Autodesk Inventor part; units mm, degrees
(part 2 of 6)
  line L866 (-45.2872, 131.2388) -> (-45.0362, 131.5916)
  line L867 (-45.0362, 131.5916) -> (-44.769, 131.9317)
  line L868 (-44.769, 131.9317) -> (-44.4862, 132.2582)
  line L869 (-44.4862, 132.2582) -> (-44.1882, 132.5707)
  line L870 (-44.1882, 132.5707) -> (-43.8757, 132.8687)
  line L871 (-43.8757, 132.8687) -> (-43.5491, 133.1516)
  line L872 (-43.5491, 133.1516) -> (-43.2091, 133.4189)
  line L873 (-43.2091, 133.4189) -> (-42.8561, 133.6697)
  line L874 (-42.8561, 133.6697) -> (-42.4911, 133.904)
  line L875 (-42.4911, 133.904) -> (-42.1142, 134.1207)
  line L876 (-42.1142, 134.1207) -> (-41.7261, 134.3194)
  line L877 (-41.7261, 134.3194) -> (-41.3274, 134.4996)
  line L878 (-41.3274, 134.4996) -> (-40.9188, 134.6609)
  line L879 (-40.9188, 134.6609) -> (-40.5005, 134.8021)
  line L880 (-40.5005, 134.8021) -> (-40.0735, 134.9234)
  line L881 (-40.0735, 134.9234) -> (-39.6381, 135.024)
  line L882 (-39.6381, 135.024) -> (-39.1949, 135.1032)
  line L883 (-39.1949, 135.1032) -> (-38.7444, 135.1604)
  line L884 (-38.7444, 135.1604) -> (-38.2874, 135.1952)
  line L885 (-38.2874, 135.1952) -> (-37.8242, 135.2069)
  line L886 (-37.8242, 135.2069) -> (-37.361, 135.1952)
  line L887 (-37.361, 135.1952) -> (-36.904, 135.1604)
  line L888 (-36.904, 135.1604) -> (-36.4536, 135.1032)
  line L889 (-36.4536, 135.1032) -> (-36.0104, 135.024)
  line L890 (-36.0104, 135.024) -> (-35.5749, 134.9234)
  line L891 (-35.5749, 134.9234) -> (-35.1479, 134.8021)
  line L892 (-35.1479, 134.8021) -> (-34.7297, 134.6609)
  line L893 (-34.7297, 134.6609) -> (-34.3211, 134.4996)
  line L894 (-34.3211, 134.4996) -> (-33.9223, 134.3194)
  line L895 (-33.9223, 134.3194) -> (-33.5342, 134.1207)
  line L896 (-33.5342, 134.1207) -> (-33.1573, 133.904)
  line L897 (-33.1573, 133.904) -> (-32.7923, 133.6697)
  line L898 (-32.7923, 133.6697) -> (-32.4394, 133.4189)
  line L899 (-32.4394, 133.4189) -> (-32.0993, 133.1516)
  line L900 (-32.0993, 133.1516) -> (-31.7729, 132.8687)
  line L901 (-31.7729, 132.8687) -> (-31.4603, 132.5707)
  line L902 (-31.4603, 132.5707) -> (-31.1623, 132.2582)
  line L903 (-31.1623, 132.2582) -> (-30.8794, 131.9317)
  line L904 (-30.8794, 131.9317) -> (-30.6123, 131.5916)
  line L905 (-30.6123, 131.5916) -> (-30.3613, 131.2388)
  line L906 (-30.3613, 131.2388) -> (-30.1272, 130.8737)
  line L907 (-30.1272, 130.8737) -> (-29.9105, 130.4968)
  line L908 (-29.9105, 130.4968) -> (-29.7117, 130.1089)
  line L909 (-29.7117, 130.1089) -> (-29.5315, 129.7099)
  line L910 (-29.5315, 129.7099) -> (-29.3703, 129.3013)
  line L911 (-29.3703, 129.3013) -> (-29.2289, 128.8831)
  line L912 (-29.2289, 128.8831) -> (-29.1076, 128.4559)
  line L913 (-29.1076, 128.4559) -> (-29.007, 128.0208)
  line L914 (-29.007, 128.0208) -> (-28.928, 127.5774)
  line L915 (-28.928, 127.5774) -> (-28.8708, 127.1271)
  line L916 (-28.8708, 127.1271) -> (-28.836, 126.67)
  line L917 (-28.836, 126.67) -> (-28.8243, 126.2069)
  line L918 (-28.8243, 126.2069) -> (-28.836, 125.7436)
  line L919 (-28.836, 125.7436) -> (-28.8708, 125.2868)
  line L920 (-28.8708, 125.2868) -> (-28.928, 124.8361)
  line L921 (-28.928, 124.8361) -> (-29.007, 124.3931)
  line L922 (-29.007, 124.3931) -> (-29.1076, 123.9576)
  line L923 (-29.1076, 123.9576) -> (-29.2289, 123.5304)
  line L924 (-29.2289, 123.5304) -> (-29.3703, 123.1122)
  line L925 (-29.3703, 123.1122) -> (-29.5315, 122.7036)
  line L926 (-29.5315, 122.7036) -> (-29.7117, 122.305)
  line L927 (-29.7117, 122.305) -> (-29.9105, 121.9168)
  line L928 (-29.9105, 121.9168) -> (-30.1272, 121.5399)
  line L929 (-30.1272, 121.5399) -> (-30.3613, 121.1747)
  line L930 (-30.3613, 121.1747) -> (-30.6123, 120.8219)
  line L931 (-30.6123, 120.8219) -> (-30.8794, 120.4819)
  line L932 (-30.8794, 120.4819) -> (-31.1623, 120.1553)
  line L933 (-31.1623, 120.1553) -> (-31.4603, 119.8428)
  line L934 (-31.4603, 119.8428) -> (-31.7729, 119.5448)
  line L935 (-31.7729, 119.5448) -> (-32.0993, 119.262)
  line L936 (-32.0993, 119.262) -> (-32.4394, 118.995)
  line L937 (-32.4394, 118.995) -> (-32.7923, 118.7438)
  line L938 (-32.7923, 118.7438) -> (-33.1573, 118.5099)
  line L939 (-33.1573, 118.5099) -> (-33.5342, 118.2932)
  line L940 (-33.5342, 118.2932) -> (-33.9223, 118.0944)
  line L941 (-33.9223, 118.0944) -> (-34.3211, 117.9142)
  line L942 (-34.3211, 117.9142) -> (-34.7297, 117.753)
  line L943 (-34.7297, 117.753) -> (-35.1479, 117.6114)
  line L944 (-35.1479, 117.6114) -> (-35.5749, 117.4902)
  line L945 (-35.5749, 117.4902) -> (-36.0104, 117.3896)
  line L946 (-36.0104, 117.3896) -> (-36.4536, 117.3107)
  line L947 (-36.4536, 117.3107) -> (-36.904, 117.2531)
  line L948 (-36.904, 117.2531) -> (-37.361, 117.2187)
  line L949 (-37.361, 117.2187) -> (-37.8242, 117.207)
  line L950 (-37.8242, 117.207) -> (-38.2874, 117.2187)
  line L951 (-38.2874, 117.2187) -> (-38.7444, 117.2531)
  line L952 (-38.7444, 117.2531) -> (-39.1949, 117.3107)
  line L953 (-39.1949, 117.3107) -> (-39.6381, 117.3896)
  line L954 (-39.6381, 117.3896) -> (-40.0735, 117.4902)
  line L955 (-40.0735, 117.4902) -> (-40.5005, 117.6114)
  line L956 (-40.5005, 117.6114) -> (-40.9188, 117.753)
  line L957 (-40.9188, 117.753) -> (-41.3274, 117.9142)
  line L958 (-41.3274, 117.9142) -> (-41.7261, 118.0944)
  line L959 (-41.7261, 118.0944) -> (-42.1142, 118.2932)
  line L960 (-42.1142, 118.2932) -> (-42.4911, 118.5099)
  line L961 (-42.4911, 118.5099) -> (-42.8561, 118.7438)
  line L962 (-42.8561, 118.7438) -> (-43.2091, 118.995)
  line L963 (-43.2091, 118.995) -> (-43.5491, 119.262)
  line L964 (-43.5491, 119.262) -> (-43.8757, 119.5448)
  line L965 (-43.8757, 119.5448) -> (-44.1882, 119.8428)
  line L966 (-44.1882, 119.8428) -> (-44.4862, 120.1553)
  line L967 (-44.4862, 120.1553) -> (-44.769, 120.4819)
  line L968 (-44.769, 120.4819) -> (-45.0362, 120.8219)
  line L969 (-45.0362, 120.8219) -> (-45.2872, 121.1747)
  line L970 (-45.2872, 121.1747) -> (-45.5213, 121.5399)
  line L971 (-45.5213, 121.5399) -> (-45.7379, 121.9168)
  line L972 (-45.7379, 121.9168) -> (-45.9367, 122.305)
  line L973 (-45.9367, 122.305) -> (-46.1169, 122.7036)
  line L974 (-46.1169, 122.7036) -> (-46.2781, 123.1122)
  line L975 (-46.2781, 123.1122) -> (-46.4196, 123.5304)
  line L976 (-46.4196, 123.5304) -> (-46.5408, 123.9576)
  line L977 (-46.5408, 123.9576) -> (-46.6414, 124.3931)
  line L978 (-46.6414, 124.3931) -> (-46.7205, 124.8361)
  line L979 (-46.7205, 124.8361) -> (-46.7777, 125.2868)
  line L980 (-46.7777, 125.2868) -> (-46.8125, 125.7436)
  line L981 (-46.8125, 125.7436) -> (-46.8242, 126.2069)
  line L982 (-46.8338, 98.1969) -> (-46.8221, 98.66)
  line L983 (-46.8221, 98.66) -> (-46.7873, 99.1171)
  line L984 (-46.7873, 99.1171) -> (-46.7301, 99.5674)
  line L985 (-46.7301, 99.5674) -> (-46.6511, 100.0108)
  line L986 (-46.6511, 100.0108) -> (-46.5505, 100.4462)
  line L987 (-46.5505, 100.4462) -> (-46.4292, 100.8731)
  line L988 (-46.4292, 100.8731) -> (-46.2878, 101.2913)
  line L989 (-46.2878, 101.2913) -> (-46.1266, 101.6999)
  line L990 (-46.1266, 101.6999) -> (-45.9464, 102.0988)
  line L991 (-45.9464, 102.0988) -> (-45.7476, 102.4868)
  line L992 (-45.7476, 102.4868) -> (-45.5309, 102.8637)
  line L993 (-45.5309, 102.8637) -> (-45.2968, 103.2288)
  line L994 (-45.2968, 103.2288) -> (-45.0458, 103.5816)
  line L995 (-45.0458, 103.5816) -> (-44.7787, 103.9216)
  line L996 (-44.7787, 103.9216) -> (-44.4958, 104.2482)
  line L997 (-44.4958, 104.2482) -> (-44.1978, 104.5607)
  line L998 (-44.1978, 104.5607) -> (-43.8852, 104.8587)
  line L999 (-43.8852, 104.8587) -> (-43.5588, 105.1416)
  line L1000 (-43.5588, 105.1416) -> (-43.2187, 105.4089)
  line L1001 (-43.2187, 105.4089) -> (-42.8658, 105.6597)
  line L1002 (-42.8658, 105.6597) -> (-42.5008, 105.894)
  line L1003 (-42.5008, 105.894) -> (-42.1239, 106.1107)
  line L1004 (-42.1239, 106.1107) -> (-41.7358, 106.3094)
  line L1005 (-41.7358, 106.3094) -> (-41.337, 106.4896)
  line L1006 (-41.337, 106.4896) -> (-40.9284, 106.6509)
  line L1007 (-40.9284, 106.6509) -> (-40.5102, 106.7921)
  line L1008 (-40.5102, 106.7921) -> (-40.0832, 106.9134)
  line L1009 (-40.0832, 106.9134) -> (-39.6477, 107.014)
  line L1010 (-39.6477, 107.014) -> (-39.2045, 107.0932)
  line L1011 (-39.2045, 107.0932) -> (-38.7541, 107.1504)
  line L1012 (-38.7541, 107.1504) -> (-38.2971, 107.1852)
  line L1013 (-38.2971, 107.1852) -> (-37.8339, 107.1969)
  line L1014 (-37.8339, 107.1969) -> (-37.3707, 107.1852)
  line L1015 (-37.3707, 107.1852) -> (-36.9137, 107.1504)
  line L1016 (-36.9137, 107.1504) -> (-36.4632, 107.0932)
  line L1017 (-36.4632, 107.0932) -> (-36.02, 107.014)
  line L1018 (-36.02, 107.014) -> (-35.5846, 106.9134)
  line L1019 (-35.5846, 106.9134) -> (-35.1575, 106.7921)
  line L1020 (-35.1575, 106.7921) -> (-34.7393, 106.6509)
  line L1021 (-34.7393, 106.6509) -> (-34.3307, 106.4896)
  line L1022 (-34.3307, 106.4896) -> (-33.932, 106.3094)
  line L1023 (-33.932, 106.3094) -> (-33.5439, 106.1107)
  line L1024 (-33.5439, 106.1107) -> (-33.167, 105.894)
  line L1025 (-33.167, 105.894) -> (-32.8018, 105.6597)
  line L1026 (-32.8018, 105.6597) -> (-32.449, 105.4089)
  line L1027 (-32.449, 105.4089) -> (-32.109, 105.1416)
  line L1028 (-32.109, 105.1416) -> (-31.7824, 104.8587)
  line L1029 (-31.7824, 104.8587) -> (-31.4699, 104.5607)
  line L1030 (-31.4699, 104.5607) -> (-31.1719, 104.2482)
  line L1031 (-31.1719, 104.2482) -> (-30.8891, 103.9216)
  line L1032 (-30.8891, 103.9216) -> (-30.6219, 103.5816)
  line L1033 (-30.6219, 103.5816) -> (-30.3709, 103.2288)
  line L1034 (-30.3709, 103.2288) -> (-30.1368, 102.8637)
  line L1035 (-30.1368, 102.8637) -> (-29.9201, 102.4868)
  line L1036 (-29.9201, 102.4868) -> (-29.7214, 102.0988)
  line L1037 (-29.7214, 102.0988) -> (-29.5412, 101.6999)
  line L1038 (-29.5412, 101.6999) -> (-29.3799, 101.2913)
  line L1039 (-29.3799, 101.2913) -> (-29.2385, 100.8731)
  line L1040 (-29.2385, 100.8731) -> (-29.1173, 100.4462)
  line L1041 (-29.1173, 100.4462) -> (-29.0167, 100.0108)
  line L1042 (-29.0167, 100.0108) -> (-28.9376, 99.5674)
  line L1043 (-28.9376, 99.5674) -> (-28.8802, 99.1171)
  line L1044 (-28.8802, 99.1171) -> (-28.8456, 98.66)
  line L1045 (-28.8456, 98.66) -> (-28.8339, 98.1969)
  line L1046 (-28.8339, 98.1969) -> (-28.8456, 97.7336)
  line L1047 (-28.8456, 97.7336) -> (-28.8802, 97.2767)
  line L1048 (-28.8802, 97.2767) -> (-28.9376, 96.8261)
  line L1049 (-28.9376, 96.8261) -> (-29.0167, 96.3831)
  line L1050 (-29.0167, 96.3831) -> (-29.1173, 95.9476)
  line L1051 (-29.1173, 95.9476) -> (-29.2385, 95.5204)
  line L1052 (-29.2385, 95.5204) -> (-29.3799, 95.1022)
  line L1053 (-29.3799, 95.1022) -> (-29.5412, 94.6936)
  line L1054 (-29.5412, 94.6936) -> (-29.7214, 94.295)
  line L1055 (-29.7214, 94.295) -> (-29.9201, 93.9068)
  line L1056 (-29.9201, 93.9068) -> (-30.1368, 93.5299)
  line L1057 (-30.1368, 93.5299) -> (-30.3709, 93.1647)
  line L1058 (-30.3709, 93.1647) -> (-30.6219, 92.8119)
  line L1059 (-30.6219, 92.8119) -> (-30.8891, 92.4719)
  line L1060 (-30.8891, 92.4719) -> (-31.1719, 92.1453)
  line L1061 (-31.1719, 92.1453) -> (-31.4699, 91.8328)
  line L1062 (-31.4699, 91.8328) -> (-31.7824, 91.5348)
  line L1063 (-31.7824, 91.5348) -> (-32.109, 91.252)
  line L1064 (-32.109, 91.252) -> (-32.449, 90.985)
  line L1065 (-32.449, 90.985) -> (-32.8018, 90.7338)
  line L1066 (-32.8018, 90.7338) -> (-33.167, 90.4999)
  line L1067 (-33.167, 90.4999) -> (-33.5439, 90.2832)
  line L1068 (-33.5439, 90.2832) -> (-33.932, 90.0844)
  line L1069 (-33.932, 90.0844) -> (-34.3307, 89.9042)
  line L1070 (-34.3307, 89.9042) -> (-34.7393, 89.743)
  line L1071 (-34.7393, 89.743) -> (-35.1575, 89.6014)
  line L1072 (-35.1575, 89.6014) -> (-35.5846, 89.4802)
  line L1073 (-35.5846, 89.4802) -> (-36.02, 89.3796)
  line L1074 (-36.02, 89.3796) -> (-36.4632, 89.3007)
  line L1075 (-36.4632, 89.3007) -> (-36.9137, 89.2431)
  line L1076 (-36.9137, 89.2431) -> (-37.3707, 89.2087)
  line L1077 (-37.3707, 89.2087) -> (-37.8339, 89.197)
  line L1078 (-37.8339, 89.197) -> (-38.2971, 89.2087)
  line L1079 (-38.2971, 89.2087) -> (-38.7541, 89.2431)
  line L1080 (-38.7541, 89.2431) -> (-39.2045, 89.3007)
  line L1081 (-39.2045, 89.3007) -> (-39.6477, 89.3796)
  line L1082 (-39.6477, 89.3796) -> (-40.0832, 89.4802)
  line L1083 (-40.0832, 89.4802) -> (-40.5102, 89.6014)
  line L1084 (-40.5102, 89.6014) -> (-40.9284, 89.743)
  line L1085 (-40.9284, 89.743) -> (-41.337, 89.9042)
  line L1086 (-41.337, 89.9042) -> (-41.7358, 90.0844)
  line L1087 (-41.7358, 90.0844) -> (-42.1239, 90.2832)
  line L1088 (-42.1239, 90.2832) -> (-42.5008, 90.4999)
  line L1089 (-42.5008, 90.4999) -> (-42.8658, 90.7338)
  line L1090 (-42.8658, 90.7338) -> (-43.2187, 90.985)
  line L1091 (-43.2187, 90.985) -> (-43.5588, 91.252)
  line L1092 (-43.5588, 91.252) -> (-43.8852, 91.5348)
  line L1093 (-43.8852, 91.5348) -> (-44.1978, 91.8328)
  line L1094 (-44.1978, 91.8328) -> (-44.4958, 92.1453)
  line L1095 (-44.4958, 92.1453) -> (-44.7787, 92.4719)
  line L1096 (-44.7787, 92.4719) -> (-45.0458, 92.8119)
  line L1097 (-45.0458, 92.8119) -> (-45.2968, 93.1647)
  line L1098 (-45.2968, 93.1647) -> (-45.5309, 93.5299)
  line L1099 (-45.5309, 93.5299) -> (-45.7476, 93.9068)
  line L1100 (-45.7476, 93.9068) -> (-45.9464, 94.295)
  line L1101 (-45.9464, 94.295) -> (-46.1266, 94.6936)
  line L1102 (-46.1266, 94.6936) -> (-46.2878, 95.1022)
  line L1103 (-46.2878, 95.1022) -> (-46.4292, 95.5204)
  line L1104 (-46.4292, 95.5204) -> (-46.5505, 95.9476)
  line L1105 (-46.5505, 95.9476) -> (-46.6511, 96.3831)
  line L1106 (-46.6511, 96.3831) -> (-46.7301, 96.8261)
  line L1107 (-46.7301, 96.8261) -> (-46.7873, 97.2767)
  line L1108 (-46.7873, 97.2767) -> (-46.8221, 97.7336)
  line L1109 (-46.8221, 97.7336) -> (-46.8338, 98.1969)
  line L1110 (-3.6981, 170.452) -> (-3.6749, 170.912)
  line L1111 (-3.6749, 170.912) -> (-3.6067, 171.3589)
  line L1112 (-3.6067, 171.3589) -> (-3.4957, 171.7902)
  line L1113 (-3.4957, 171.7902) -> (-3.3445, 172.2036)
  line L1114 (-3.3445, 172.2036) -> (-3.155, 172.5969)
  line L1115 (-3.155, 172.5969) -> (-2.9295, 172.9679)
  line L1116 (-2.9295, 172.9679) -> (-2.6705, 173.3143)
  line L1117 (-2.6705, 173.3143) -> (-2.38, 173.634)
  line L1118 (-2.38, 173.634) -> (-2.0605, 173.9244)
  line L1119 (-2.0605, 173.9244) -> (-1.7141, 174.1835)
  line L1120 (-1.7141, 174.1835) -> (-1.3431, 174.4088)
  line L1121 (-1.3431, 174.4088) -> (-0.9496, 174.5983)
  line L1122 (-0.9496, 174.5983) -> (-0.5362, 174.7497)
  line L1123 (-0.5362, 174.7497) -> (-0.1051, 174.8605)
  line L1124 (-0.1051, 174.8605) -> (0.3418, 174.9287)
  line L1125 (0.3418, 174.9287) -> (0.8018, 174.9519)
  line L1126 (0.8018, 174.9519) -> (1.2619, 174.9287)
  line L1127 (1.2619, 174.9287) -> (1.7088, 174.8605)
  line L1128 (1.7088, 174.8605) -> (2.1401, 174.7497)
  line L1129 (2.1401, 174.7497) -> (2.5535, 174.5983)
  line L1130 (2.5535, 174.5983) -> (2.9469, 174.4088)
  line L1131 (2.9469, 174.4088) -> (3.318, 174.1835)
  line L1132 (3.318, 174.1835) -> (3.6644, 173.9244)
  line L1133 (3.6644, 173.9244) -> (3.9839, 173.634)
  line L1134 (3.9839, 173.634) -> (4.2743, 173.3143)
  line L1135 (4.2743, 173.3143) -> (4.5334, 172.9679)
  line L1136 (4.5334, 172.9679) -> (4.7587, 172.5969)
  line L1137 (4.7587, 172.5969) -> (4.9482, 172.2036)
  line L1138 (4.9482, 172.2036) -> (5.0996, 171.7902)
  line L1139 (5.0996, 171.7902) -> (5.2105, 171.3589)
  line L1140 (5.2105, 171.3589) -> (5.2787, 170.912)
  line L1141 (5.2787, 170.912) -> (5.3018, 170.452)
  line L1142 (5.3018, 170.452) -> (5.2787, 169.9919)
  line L1143 (5.2787, 169.9919) -> (5.2105, 169.545)
  line L1144 (5.2105, 169.545) -> (5.0996, 169.1139)
  line L1145 (5.0996, 169.1139) -> (4.9482, 168.7003)
  line L1146 (4.9482, 168.7003) -> (4.7587, 168.307)
  line L1147 (4.7587, 168.307) -> (4.5334, 167.936)
  line L1148 (4.5334, 167.936) -> (4.2743, 167.5896)
  line L1149 (4.2743, 167.5896) -> (3.9839, 167.2701)
  line L1150 (3.9839, 167.2701) -> (3.6644, 166.9795)
  line L1151 (3.6644, 166.9795) -> (3.318, 166.7206)
  line L1152 (3.318, 166.7206) -> (2.9469, 166.4951)
  line L1153 (2.9469, 166.4951) -> (2.5535, 166.3056)
  line L1154 (2.5535, 166.3056) -> (2.1401, 166.1542)
  line L1155 (2.1401, 166.1542) -> (1.7088, 166.0434)
  line L1156 (1.7088, 166.0434) -> (1.2619, 165.9752)
  line L1157 (1.2619, 165.9752) -> (0.8018, 165.952)
  line L1158 (0.8018, 165.952) -> (0.3418, 165.9752)
  line L1159 (0.3418, 165.9752) -> (-0.1051, 166.0434)
  line L1160 (-0.1051, 166.0434) -> (-0.5362, 166.1542)
  line L1161 (-0.5362, 166.1542) -> (-0.9496, 166.3056)
  line L1162 (-0.9496, 166.3056) -> (-1.3431, 166.4951)
  line L1163 (-1.3431, 166.4951) -> (-1.7141, 166.7206)
  line L1164 (-1.7141, 166.7206) -> (-2.0605, 166.9795)
  line L1165 (-2.0605, 166.9795) -> (-2.38, 167.2701)
  line L1166 (-2.38, 167.2701) -> (-2.6705, 167.5896)
  line L1167 (-2.6705, 167.5896) -> (-2.9295, 167.936)
  line L1168 (-2.9295, 167.936) -> (-3.155, 168.307)
  line L1169 (-3.155, 168.307) -> (-3.3445, 168.7003)
  line L1170 (-3.3445, 168.7003) -> (-3.4957, 169.1139)
  line L1171 (-3.4957, 169.1139) -> (-3.6067, 169.545)
  line L1172 (-3.6067, 169.545) -> (-3.6749, 169.9919)
  line L1173 (-3.6749, 169.9919) -> (-3.6981, 170.452)
  line L1174 (-3.7014, 126.9587) -> (-3.6782, 127.4189)
  line L1175 (-3.6782, 127.4189) -> (-3.6099, 127.8658)
  line L1176 (-3.6099, 127.8658) -> (-3.499, 128.2971)
  line L1177 (-3.499, 128.2971) -> (-3.3478, 128.7105)
  line L1178 (-3.3478, 128.7105) -> (-3.1583, 129.1039)
  line L1179 (-3.1583, 129.1039) -> (-2.9328, 129.475)
  line L1180 (-2.9328, 129.475) -> (-2.6737, 129.8212)
  line L1181 (-2.6737, 129.8212) -> (-2.3833, 130.1409)
  line L1182 (-2.3833, 130.1409) -> (-2.0638, 130.4313)
  line L1183 (-2.0638, 130.4313) -> (-1.7174, 130.6904)
  line L1184 (-1.7174, 130.6904) -> (-1.3463, 130.9157)
  line L1185 (-1.3463, 130.9157) -> (-0.9529, 131.1052)
  line L1186 (-0.9529, 131.1052) -> (-0.5395, 131.2564)
  line L1187 (-0.5395, 131.2564) -> (-0.1082, 131.3673)
  line L1188 (-0.1082, 131.3673) -> (0.3385, 131.4356)
  line L1189 (0.3385, 131.4356) -> (0.7986, 131.4586)
  line L1190 (0.7986, 131.4586) -> (1.2588, 131.4356)
  line L1191 (1.2588, 131.4356) -> (1.7055, 131.3673)
  line L1192 (1.7055, 131.3673) -> (2.1368, 131.2564)
  line L1193 (2.1368, 131.2564) -> (2.5502, 131.1052)
  line L1194 (2.5502, 131.1052) -> (2.9437, 130.9157)
  line L1195 (2.9437, 130.9157) -> (3.3147, 130.6904)
  line L1196 (3.3147, 130.6904) -> (3.6611, 130.4313)
  line L1197 (3.6611, 130.4313) -> (3.9806, 130.1409)
  line L1198 (3.9806, 130.1409) -> (4.2711, 129.8212)
  line L1199 (4.2711, 129.8212) -> (4.5301, 129.475)
  line L1200 (4.5301, 129.475) -> (4.7556, 129.1039)
  line L1201 (4.7556, 129.1039) -> (4.9451, 128.7105)
  line L1202 (4.9451, 128.7105) -> (5.0963, 128.2971)
  line L1203 (5.0963, 128.2971) -> (5.2073, 127.8658)
  line L1204 (5.2073, 127.8658) -> (5.2755, 127.4189)
  line L1205 (5.2755, 127.4189) -> (5.2987, 126.9587)
  line L1206 (5.2987, 126.9587) -> (5.2755, 126.4987)
  line L1207 (5.2755, 126.4987) -> (5.2073, 126.0519)
  line L1208 (5.2073, 126.0519) -> (5.0963, 125.6206)
  line L1209 (5.0963, 125.6206) -> (4.9451, 125.2072)
  line L1210 (4.9451, 125.2072) -> (4.7556, 124.8137)
  line L1211 (4.7556, 124.8137) -> (4.5301, 124.4427)
  line L1212 (4.5301, 124.4427) -> (4.2711, 124.0965)
  line L1213 (4.2711, 124.0965) -> (3.9806, 123.7768)
  line L1214 (3.9806, 123.7768) -> (3.6611, 123.4863)
  line L1215 (3.6611, 123.4863) -> (3.3147, 123.2273)
  line L1216 (3.3147, 123.2273) -> (2.9437, 123.002)
  line L1217 (2.9437, 123.002) -> (2.5502, 122.8125)
  line L1218 (2.5502, 122.8125) -> (2.1368, 122.6612)
  line L1219 (2.1368, 122.6612) -> (1.7055, 122.5503)
  line L1220 (1.7055, 122.5503) -> (1.2588, 122.4821)
  line L1221 (1.2588, 122.4821) -> (0.7986, 122.4587)
  line L1222 (0.7986, 122.4587) -> (0.3385, 122.4821)
  line L1223 (0.3385, 122.4821) -> (-0.1082, 122.5503)
  line L1224 (-0.1082, 122.5503) -> (-0.5395, 122.6612)
  line L1225 (-0.5395, 122.6612) -> (-0.9529, 122.8125)
  line L1226 (-0.9529, 122.8125) -> (-1.3463, 123.002)
  line L1227 (-1.3463, 123.002) -> (-1.7174, 123.2273)
  line L1228 (-1.7174, 123.2273) -> (-2.0638, 123.4863)
  line L1229 (-2.0638, 123.4863) -> (-2.3833, 123.7768)
  line L1230 (-2.3833, 123.7768) -> (-2.6737, 124.0965)
  line L1231 (-2.6737, 124.0965) -> (-2.9328, 124.4427)
  line L1232 (-2.9328, 124.4427) -> (-3.1583, 124.8137)
  line L1233 (-3.1583, 124.8137) -> (-3.3478, 125.2072)
  line L1234 (-3.3478, 125.2072) -> (-3.499, 125.6206)
  line L1235 (-3.499, 125.6206) -> (-3.6099, 126.0519)
  line L1236 (-3.6099, 126.0519) -> (-3.6782, 126.4987)
  line L1237 (-3.6782, 126.4987) -> (-3.7014, 126.9587)
  line L1238 (-20.9892, 202.2026) -> (-20.9815, 202.5113)
  line L1239 (-20.9815, 202.5113) -> (-20.9582, 202.816)
  line L1240 (-20.9582, 202.816) -> (-20.9202, 203.1163)
  line L1241 (-20.9202, 203.1163) -> (-20.8673, 203.4119)
  line L1242 (-20.8673, 203.4119) -> (-20.7195, 203.9869)
  line L1243 (-20.7195, 203.9869) -> (-20.5178, 204.5381)
  line L1244 (-20.5178, 204.5381) -> (-20.2651, 205.0626)
  line L1245 (-20.2651, 205.0626) -> (-19.9645, 205.5573)
  line L1246 (-19.9645, 205.5573) -> (-19.6191, 206.0191)
  line L1247 (-19.6191, 206.0191) -> (-19.2319, 206.4453)
  line L1248 (-19.2319, 206.4453) -> (-18.8057, 206.8325)
  line L1249 (-18.8057, 206.8325) -> (-18.3439, 207.1779)
  line L1250 (-18.3439, 207.1779) -> (-17.8492, 207.4785)
  line L1251 (-17.8492, 207.4785) -> (-17.3247, 207.731)
  line L1252 (-17.3247, 207.731) -> (-16.7735, 207.9329)
  line L1253 (-16.7735, 207.9329) -> (-16.1985, 208.0807)
  line L1254 (-16.1985, 208.0807) -> (-15.9029, 208.1334)
  line L1255 (-15.9029, 208.1334) -> (-15.6027, 208.1716)
  line L1256 (-15.6027, 208.1716) -> (-15.2979, 208.1947)
  line L1257 (-15.2979, 208.1947) -> (-14.9893, 208.2026)
  line L1258 (-14.9893, 208.2026) -> (-14.6804, 208.1947)
  line L1259 (-14.6804, 208.1947) -> (-14.3757, 208.1716)
  line L1260 (-14.3757, 208.1716) -> (-14.0755, 208.1334)
  line L1261 (-14.0755, 208.1334) -> (-13.78, 208.0807)
  line L1262 (-13.78, 208.0807) -> (-13.2051, 207.9329)
  line L1263 (-13.2051, 207.9329) -> (-12.6538, 207.731)
  line L1264 (-12.6538, 207.731) -> (-12.1293, 207.4785)
  line L1265 (-12.1293, 207.4785) -> (-11.6346, 207.1779)
  line L1266 (-11.6346, 207.1779) -> (-11.1726, 206.8325)
  line L1267 (-11.1726, 206.8325) -> (-10.7466, 206.4453)
  line L1268 (-10.7466, 206.4453) -> (-10.3594, 206.0191)
  line L1269 (-10.3594, 206.0191) -> (-10.0139, 205.5573)
  line L1270 (-10.0139, 205.5573) -> (-9.7134, 205.0626)
  line L1271 (-9.7134, 205.0626) -> (-9.4607, 204.5381)
  line L1272 (-9.4607, 204.5381) -> (-9.259, 203.9869)
  line L1273 (-9.259, 203.9869) -> (-9.1111, 203.4119)
  line L1274 (-9.1111, 203.4119) -> (-9.0584, 203.1163)
  line L1275 (-9.0584, 203.1163) -> (-9.0201, 202.816)
  line L1276 (-9.0201, 202.816) -> (-8.997, 202.5113)
  line L1277 (-8.997, 202.5113) -> (-8.9893, 202.2026)
  line L1278 (-8.9893, 202.2026) -> (-8.997, 201.8938)
  line L1279 (-8.997, 201.8938) -> (-9.0201, 201.5891)
  line L1280 (-9.0201, 201.5891) -> (-9.0584, 201.2888)
  line L1281 (-9.0584, 201.2888) -> (-9.1111, 200.9934)
  line L1282 (-9.1111, 200.9934) -> (-9.259, 200.4184)
  line L1283 (-9.259, 200.4184) -> (-9.4607, 199.8672)
  line L1284 (-9.4607, 199.8672) -> (-9.7134, 199.3427)
  line L1285 (-9.7134, 199.3427) -> (-10.0139, 198.848)
  line L1286 (-10.0139, 198.848) -> (-10.3594, 198.386)
  line L1287 (-10.3594, 198.386) -> (-10.7466, 197.96)
  line L1288 (-10.7466, 197.96) -> (-11.1726, 197.5728)
  line L1289 (-11.1726, 197.5728) -> (-11.6346, 197.2272)
  line L1290 (-11.6346, 197.2272) -> (-12.1293, 196.9268)
  line L1291 (-12.1293, 196.9268) -> (-12.6538, 196.6741)
  line L1292 (-12.6538, 196.6741) -> (-13.2051, 196.4724)
  line L1293 (-13.2051, 196.4724) -> (-13.78, 196.3245)
  line L1294 (-13.78, 196.3245) -> (-14.0755, 196.2717)
  line L1295 (-14.0755, 196.2717) -> (-14.3757, 196.2335)
  line L1296 (-14.3757, 196.2335) -> (-14.6804, 196.2104)
  line L1297 (-14.6804, 196.2104) -> (-14.9893, 196.2027)
  line L1298 (-14.9893, 196.2027) -> (-15.2979, 196.2104)
  line L1299 (-15.2979, 196.2104) -> (-15.6027, 196.2335)
  line L1300 (-15.6027, 196.2335) -> (-15.9029, 196.2717)
  line L1301 (-15.9029, 196.2717) -> (-16.1985, 196.3245)
  line L1302 (-16.1985, 196.3245) -> (-16.7735, 196.4724)
  line L1303 (-16.7735, 196.4724) -> (-17.3247, 196.6741)
  line L1304 (-17.3247, 196.6741) -> (-17.8492, 196.9268)
  line L1305 (-17.8492, 196.9268) -> (-18.3439, 197.2272)
  line L1306 (-18.3439, 197.2272) -> (-18.8057, 197.5728)
  line L1307 (-18.8057, 197.5728) -> (-19.2319, 197.96)
  line L1308 (-19.2319, 197.96) -> (-19.6191, 198.386)
  line L1309 (-19.6191, 198.386) -> (-19.9645, 198.848)
  line L1310 (-19.9645, 198.848) -> (-20.2651, 199.3427)
  line L1311 (-20.2651, 199.3427) -> (-20.5178, 199.8672)
  line L1312 (-20.5178, 199.8672) -> (-20.7195, 200.4184)
  line L1313 (-20.7195, 200.4184) -> (-20.8673, 200.9934)
  line L1314 (-20.8673, 200.9934) -> (-20.9202, 201.2888)
  line L1315 (-20.9202, 201.2888) -> (-20.9582, 201.5891)
  line L1316 (-20.9582, 201.5891) -> (-20.9815, 201.8938)
  line L1317 (-20.9815, 201.8938) -> (-20.9892, 202.2026)
  line L1318 (-20.9892, 95.1987) -> (-20.9815, 95.5073)
  line L1319 (-20.9815, 95.5073) -> (-20.9582, 95.8119)
  line L1320 (-20.9582, 95.8119) -> (-20.9202, 96.1123)
  line L1321 (-20.9202, 96.1123) -> (-20.8673, 96.4079)
  line L1322 (-20.8673, 96.4079) -> (-20.7195, 96.9829)
  line L1323 (-20.7195, 96.9829) -> (-20.5178, 97.5341)
  line L1324 (-20.5178, 97.5341) -> (-20.2651, 98.0584)
  line L1325 (-20.2651, 98.0584) -> (-19.9645, 98.5532)
  line L1326 (-19.9645, 98.5532) -> (-19.6191, 99.0151)
  line L1327 (-19.6191, 99.0151) -> (-19.2319, 99.4413)
  line L1328 (-19.2319, 99.4413) -> (-18.8057, 99.8285)
  line L1329 (-18.8057, 99.8285) -> (-18.3439, 100.1737)
  line L1330 (-18.3439, 100.1737) -> (-17.8492, 100.4745)
  line L1331 (-17.8492, 100.4745) -> (-17.3247, 100.727)
  line L1332 (-17.3247, 100.727) -> (-16.7735, 100.9289)
  line L1333 (-16.7735, 100.9289) -> (-16.1985, 101.0767)
  line L1334 (-16.1985, 101.0767) -> (-15.9029, 101.1294)
  line L1335 (-15.9029, 101.1294) -> (-15.6027, 101.1676)
  line L1336 (-15.6027, 101.1676) -> (-15.2979, 101.1907)
  line L1337 (-15.2979, 101.1907) -> (-14.9893, 101.1986)
  line L1338 (-14.9893, 101.1986) -> (-14.6804, 101.1907)
  line L1339 (-14.6804, 101.1907) -> (-14.3757, 101.1676)
  line L1340 (-14.3757, 101.1676) -> (-14.0755, 101.1294)
  line L1341 (-14.0755, 101.1294) -> (-13.78, 101.0767)
  line L1342 (-13.78, 101.0767) -> (-13.2051, 100.9289)
  line L1343 (-13.2051, 100.9289) -> (-12.6538, 100.727)
  line L1344 (-12.6538, 100.727) -> (-12.1293, 100.4745)
  line L1345 (-12.1293, 100.4745) -> (-11.6346, 100.1737)
  line L1346 (-11.6346, 100.1737) -> (-11.1726, 99.8285)
  line L1347 (-11.1726, 99.8285) -> (-10.7466, 99.4413)
  line L1348 (-10.7466, 99.4413) -> (-10.3594, 99.0151)
  line L1349 (-10.3594, 99.0151) -> (-10.0139, 98.5532)
  line L1350 (-10.0139, 98.5532) -> (-9.7134, 98.0584)
  line L1351 (-9.7134, 98.0584) -> (-9.4607, 97.5341)
  line L1352 (-9.4607, 97.5341) -> (-9.259, 96.9829)
  line L1353 (-9.259, 96.9829) -> (-9.1111, 96.4079)
  line L1354 (-9.1111, 96.4079) -> (-9.0584, 96.1123)
  line L1355 (-9.0584, 96.1123) -> (-9.0201, 95.8119)
  line L1356 (-9.0201, 95.8119) -> (-8.997, 95.5073)
  line L1357 (-8.997, 95.5073) -> (-8.9893, 95.1987)
  line L1358 (-8.9893, 95.1987) -> (-8.997, 94.8896)
  line L1359 (-8.997, 94.8896) -> (-9.0201, 94.5851)
  line L1360 (-9.0201, 94.5851) -> (-9.0584, 94.2847)
  line L1361 (-9.0584, 94.2847) -> (-9.1111, 93.9894)
  line L1362 (-9.1111, 93.9894) -> (-9.259, 93.4145)
  line L1363 (-9.259, 93.4145) -> (-9.4607, 92.8632)
  line L1364 (-9.4607, 92.8632) -> (-9.7134, 92.3385)
  line L1365 (-9.7134, 92.3385) -> (-10.0139, 91.8438)
  line L1366 (-10.0139, 91.8438) -> (-10.3594, 91.3818)
  line L1367 (-10.3594, 91.3818) -> (-10.7466, 90.956)
  line L1368 (-10.7466, 90.956) -> (-11.1726, 90.5688)
  line L1369 (-11.1726, 90.5688) -> (-11.6346, 90.2233)
  line L1370 (-11.6346, 90.2233) -> (-12.1293, 89.9228)
  line L1371 (-12.1293, 89.9228) -> (-12.6538, 89.67)
  line L1372 (-12.6538, 89.67) -> (-13.2051, 89.4684)
  line L1373 (-13.2051, 89.4684) -> (-13.78, 89.3203)
  line L1374 (-13.78, 89.3203) -> (-14.0755, 89.2676)
  line L1375 (-14.0755, 89.2676) -> (-14.3757, 89.2294)
  line L1376 (-14.3757, 89.2294) -> (-14.6804, 89.2063)
  line L1377 (-14.6804, 89.2063) -> (-14.9893, 89.1987)
  line L1378 (-14.9893, 89.1987) -> (-15.2979, 89.2063)
  line L1379 (-15.2979, 89.2063) -> (-15.6027, 89.2294)
  line L1380 (-15.6027, 89.2294) -> (-15.9029, 89.2676)
  line L1381 (-15.9029, 89.2676) -> (-16.1985, 89.3203)
  line L1382 (-16.1985, 89.3203) -> (-16.7735, 89.4684)
  line L1383 (-16.7735, 89.4684) -> (-17.3247, 89.67)
  line L1384 (-17.3247, 89.67) -> (-17.8492, 89.9228)
  line L1385 (-17.8492, 89.9228) -> (-18.3439, 90.2233)
  line L1386 (-18.3439, 90.2233) -> (-18.8057, 90.5688)
  line L1387 (-18.8057, 90.5688) -> (-19.2319, 90.956)
  line L1388 (-19.2319, 90.956) -> (-19.6191, 91.3818)
  line L1389 (-19.6191, 91.3818) -> (-19.9645, 91.8438)
  line L1390 (-19.9645, 91.8438) -> (-20.2651, 92.3385)
  line L1391 (-20.2651, 92.3385) -> (-20.5178, 92.8632)
  line L1392 (-20.5178, 92.8632) -> (-20.7195, 93.4145)
  line L1393 (-20.7195, 93.4145) -> (-20.8673, 93.9894)
  line L1394 (-20.8673, 93.9894) -> (-20.9202, 94.2847)
  line L1395 (-20.9202, 94.2847) -> (-20.9582, 94.5851)
  line L1396 (-20.9582, 94.5851) -> (-20.9815, 94.8896)
  line L1397 (-20.9815, 94.8896) -> (-20.9892, 95.1987)
  spline S3 degree 3 poles (-27.8908, 137.7318) (-27.8908, 135.5228) (-26.0999, 133.7317) (-23.8907, 133.7317) knots 0 0 0 0 1 1 1 1
  line L1398 (-27.8908, 137.7318) -> (-27.8908, 135.5228) construction
  line L1399 (-27.8908, 135.5228) -> (-26.0999, 133.7317) construction
  line L1400 (-26.0999, 133.7317) -> (-23.8907, 133.7317) construction
  line L1401 (-23.8907, 133.7317) -> (-5.8918, 133.7317)
  spline S4 degree 3 poles (-5.8918, 133.7317) (-3.6826, 133.7317) (-1.8917, 135.5228) (-1.8917, 137.7318) knots 2 2 2 2 3 3 3 3
  line L1402 (-5.8918, 133.7317) -> (-3.6826, 133.7317) construction
  line L1403 (-3.6826, 133.7317) -> (-1.8917, 135.5228) construction
  line L1404 (-1.8917, 135.5228) -> (-1.8917, 137.7318) construction
  line L1405 (-1.8917, 137.7318) -> (-1.8917, 159.7319)
  spline S5 degree 3 poles (-1.8917, 159.7319) (-1.8917, 161.941) (-3.6826, 163.7318) (-5.8918, 163.7318) knots 4 4 4 4 5 5 5 5
  line L1406 (-1.8917, 159.7319) -> (-1.8917, 161.941) construction
  line L1407 (-1.8917, 161.941) -> (-3.6826, 163.7318) construction
  line L1408 (-3.6826, 163.7318) -> (-5.8918, 163.7318) construction
  line L1409 (-5.8918, 163.7318) -> (-23.8907, 163.7318)
  spline S6 degree 3 poles (-23.8907, 163.7318) (-26.0999, 163.7318) (-27.8908, 161.941) (-27.8908, 159.7319) knots 6 6 6 6 7 7 7 7
  line L1410 (-23.8907, 163.7318) -> (-26.0999, 163.7318) construction
  line L1411 (-26.0999, 163.7318) -> (-27.8908, 161.941) construction
  line L1412 (-27.8908, 161.941) -> (-27.8908, 159.7319) construction
  line L1413 (-27.8908, 159.7319) -> (-27.8908, 137.7318)
  line L1414 (222.3778, 185.1978) -> (222.3919, 185.4789)
  line L1415 (222.3919, 185.4789) -> (222.4336, 185.752)
  line L1416 (222.4336, 185.752) -> (222.5015, 186.0155)
  line L1417 (222.5015, 186.0155) -> (222.5938, 186.2682)
  line L1418 (222.5938, 186.2682) -> (222.7096, 186.5087)
  line L1419 (222.7096, 186.5087) -> (222.8474, 186.7354)
  line L1420 (222.8474, 186.7354) -> (223.0059, 186.9471)
  line L1421 (223.0059, 186.9471) -> (223.1833, 187.1424)
  line L1422 (223.1833, 187.1424) -> (223.3786, 187.3198)
  line L1423 (223.3786, 187.3198) -> (223.5901, 187.4781)
  line L1424 (223.5901, 187.4781) -> (223.8168, 187.6159)
  line L1425 (223.8168, 187.6159) -> (224.0573, 187.7317)
  line L1426 (224.0573, 187.7317) -> (224.3102, 187.8242)
  line L1427 (224.3102, 187.8242) -> (224.5737, 187.8919)
  line L1428 (224.5737, 187.8919) -> (224.8466, 187.9336)
  line L1429 (224.8466, 187.9336) -> (225.1277, 187.9479)
  line L1430 (225.1277, 187.9479) -> (225.4088, 187.9336)
  line L1431 (225.4088, 187.9336) -> (225.682, 187.8919)
  line L1432 (225.682, 187.8919) -> (225.9456, 187.8242)
  line L1433 (225.9456, 187.8242) -> (226.1981, 187.7317)
  line L1434 (226.1981, 187.7317) -> (226.4385, 187.6159)
  line L1435 (226.4385, 187.6159) -> (226.6652, 187.4781)
  line L1436 (226.6652, 187.4781) -> (226.8771, 187.3198)
  line L1437 (226.8771, 187.3198) -> (227.0724, 187.1424)
  line L1438 (227.0724, 187.1424) -> (227.2499, 186.9471)
  line L1439 (227.2499, 186.9471) -> (227.408, 186.7354)
  line L1440 (227.408, 186.7354) -> (227.5458, 186.5087)
  line L1441 (227.5458, 186.5087) -> (227.6616, 186.2682)
  line L1442 (227.6616, 186.2682) -> (227.7542, 186.0155)
  line L1443 (227.7542, 186.0155) -> (227.8218, 185.752)
  line L1444 (227.8218, 185.752) -> (227.8634, 185.4789)
  line L1445 (227.8634, 185.4789) -> (227.8779, 185.1978)
  line L1446 (227.8779, 185.1978) -> (227.8634, 184.9167)
  line L1447 (227.8634, 184.9167) -> (227.8218, 184.6437)
  line L1448 (227.8218, 184.6437) -> (227.7542, 184.3801)
  line L1449 (227.7542, 184.3801) -> (227.6616, 184.1274)
  line L1450 (227.6616, 184.1274) -> (227.5458, 183.887)
  line L1451 (227.5458, 183.887) -> (227.408, 183.6603)
  line L1452 (227.408, 183.6603) -> (227.2499, 183.4486)
  line L1453 (227.2499, 183.4486) -> (227.0724, 183.2532)
  line L1454 (227.0724, 183.2532) -> (226.8771, 183.0758)
  line L1455 (226.8771, 183.0758) -> (226.6652, 182.9175)
  line L1456 (226.6652, 182.9175) -> (226.4385, 182.7797)
  line L1457 (226.4385, 182.7797) -> (226.1981, 182.664)
  line L1458 (226.1981, 182.664) -> (225.9456, 182.5715)
  line L1459 (225.9456, 182.5715) -> (225.682, 182.5038)
  line L1460 (225.682, 182.5038) -> (225.4088, 182.4621)
  line L1461 (225.4088, 182.4621) -> (225.1277, 182.4478)
  line L1462 (225.1277, 182.4478) -> (224.8466, 182.4621)
  line L1463 (224.8466, 182.4621) -> (224.5737, 182.5038)
  line L1464 (224.5737, 182.5038) -> (224.3102, 182.5715)
  line L1465 (224.3102, 182.5715) -> (224.0573, 182.664)
  line L1466 (224.0573, 182.664) -> (223.8168, 182.7797)
  line L1467 (223.8168, 182.7797) -> (223.5901, 182.9175)
  line L1468 (223.5901, 182.9175) -> (223.3786, 183.0758)
  line L1469 (223.3786, 183.0758) -> (223.1833, 183.2532)
  line L1470 (223.1833, 183.2532) -> (223.0059, 183.4486)
  line L1471 (223.0059, 183.4486) -> (222.8474, 183.6603)
  line L1472 (222.8474, 183.6603) -> (222.7096, 183.887)
  line L1473 (222.7096, 183.887) -> (222.5938, 184.1274)
  line L1474 (222.5938, 184.1274) -> (222.5015, 184.3801)
  line L1475 (222.5015, 184.3801) -> (222.4336, 184.6437)
  line L1476 (222.4336, 184.6437) -> (222.3919, 184.9167)
  line L1477 (222.3919, 184.9167) -> (222.3778, 185.1978)
  line L1478 (222.3778, 112.1988) -> (222.3919, 112.48)
  line L1479 (222.3919, 112.48) -> (222.4336, 112.7532)
  line L1480 (222.4336, 112.7532) -> (222.5015, 113.0167)
  line L1481 (222.5015, 113.0167) -> (222.5938, 113.2692)
  line L1482 (222.5938, 113.2692) -> (222.7096, 113.5097)
  line L1483 (222.7096, 113.5097) -> (222.8474, 113.7364)
  line L1484 (222.8474, 113.7364) -> (223.0059, 113.9479)
  line L1485 (223.0059, 113.9479) -> (223.1833, 114.1432)
  line L1486 (223.1833, 114.1432) -> (223.3786, 114.321)
  line L1487 (223.3786, 114.321) -> (223.5901, 114.4791)
  line L1488 (223.5901, 114.4791) -> (223.8168, 114.6169)
  line L1489 (223.8168, 114.6169) -> (224.0573, 114.7327)
  line L1490 (224.0573, 114.7327) -> (224.3102, 114.825)
  line L1491 (224.3102, 114.825) -> (224.5737, 114.8929)
  line L1492 (224.5737, 114.8929) -> (224.8466, 114.9346)
  line L1493 (224.8466, 114.9346) -> (225.1277, 114.9487)
  line L1494 (225.1277, 114.9487) -> (225.4088, 114.9346)
  line L1495 (225.4088, 114.9346) -> (225.682, 114.8929)
  line L1496 (225.682, 114.8929) -> (225.9456, 114.825)
  line L1497 (225.9456, 114.825) -> (226.1981, 114.7327)
  line L1498 (226.1981, 114.7327) -> (226.4385, 114.6169)
  line L1499 (226.4385, 114.6169) -> (226.6652, 114.4791)
  line L1500 (226.6652, 114.4791) -> (226.8771, 114.321)
  line L1501 (226.8771, 114.321) -> (227.0724, 114.1432)
  line L1502 (227.0724, 114.1432) -> (227.2499, 113.9479)
  line L1503 (227.2499, 113.9479) -> (227.408, 113.7364)
  line L1504 (227.408, 113.7364) -> (227.5458, 113.5097)
  line L1505 (227.5458, 113.5097) -> (227.6616, 113.2692)
  line L1506 (227.6616, 113.2692) -> (227.7542, 113.0167)
  line L1507 (227.7542, 113.0167) -> (227.8218, 112.7532)
  line L1508 (227.8218, 112.7532) -> (227.8634, 112.48)
  line L1509 (227.8634, 112.48) -> (227.8779, 112.1988)
  line L1510 (227.8779, 112.1988) -> (227.8634, 111.9177)
  line L1511 (227.8634, 111.9177) -> (227.8218, 111.6445)
  line L1512 (227.8218, 111.6445) -> (227.7542, 111.381)
  line L1513 (227.7542, 111.381) -> (227.6616, 111.1284)
  line L1514 (227.6616, 111.1284) -> (227.5458, 110.888)
  line L1515 (227.5458, 110.888) -> (227.408, 110.6613)
  line L1516 (227.408, 110.6613) -> (227.2499, 110.4494)
  line L1517 (227.2499, 110.4494) -> (227.0724, 110.2544)
  line L1518 (227.0724, 110.2544) -> (226.8771, 110.0767)
  line L1519 (226.8771, 110.0767) -> (226.6652, 109.9185)
  line L1520 (226.6652, 109.9185) -> (226.4385, 109.7807)
  line L1521 (226.4385, 109.7807) -> (226.1981, 109.665)
  line L1522 (226.1981, 109.665) -> (225.9456, 109.5726)
  line L1523 (225.9456, 109.5726) -> (225.682, 109.5048)
  line L1524 (225.682, 109.5048) -> (225.4088, 109.4631)
  line L1525 (225.4088, 109.4631) -> (225.1277, 109.449)
  line L1526 (225.1277, 109.449) -> (224.8466, 109.4631)
  line L1527 (224.8466, 109.4631) -> (224.5737, 109.5048)
  line L1528 (224.5737, 109.5048) -> (224.3102, 109.5726)
  line L1529 (224.3102, 109.5726) -> (224.0573, 109.665)
  line L1530 (224.0573, 109.665) -> (223.8168, 109.7807)
  line L1531 (223.8168, 109.7807) -> (223.5901, 109.9185)
  line L1532 (223.5901, 109.9185) -> (223.3786, 110.0767)
  line L1533 (223.3786, 110.0767) -> (223.1833, 110.2544)
  line L1534 (223.1833, 110.2544) -> (223.0059, 110.4494)
  line L1535 (223.0059, 110.4494) -> (222.8474, 110.6613)
  line L1536 (222.8474, 110.6613) -> (222.7096, 110.888)
  line L1537 (222.7096, 110.888) -> (222.5938, 111.1284)
  line L1538 (222.5938, 111.1284) -> (222.5015, 111.381)
  line L1539 (222.5015, 111.381) -> (222.4336, 111.6445)
  line L1540 (222.4336, 111.6445) -> (222.3919, 111.9177)
  line L1541 (222.3919, 111.9177) -> (222.3778, 112.1988)
  line L1542 (-17.6222, 185.1949) -> (-17.6081, 185.476)
  line L1543 (-17.6081, 185.476) -> (-17.5664, 185.749)
  line L1544 (-17.5664, 185.749) -> (-17.4987, 186.0126)
  line L1545 (-17.4987, 186.0126) -> (-17.4062, 186.2653)
  line L1546 (-17.4062, 186.2653) -> (-17.2902, 186.5056)
  line L1547 (-17.2902, 186.5056) -> (-17.1526, 186.7324)
  line L1548 (-17.1526, 186.7324) -> (-16.9943, 186.9441)
  line L1549 (-16.9943, 186.9441) -> (-16.8167, 187.1393)
  line L1550 (-16.8167, 187.1393) -> (-16.6216, 187.3169)
  line L1551 (-16.6216, 187.3169) -> (-16.4099, 187.4752)
  line L1552 (-16.4099, 187.4752) -> (-16.183, 187.613)
  line L1553 (-16.183, 187.613) -> (-15.9427, 187.7288)
  line L1554 (-15.9427, 187.7288) -> (-15.69, 187.8213)
  line L1555 (-15.69, 187.8213) -> (-15.4264, 187.889)
  line L1556 (-15.4264, 187.889) -> (-15.1534, 187.9306)
  line L1557 (-15.1534, 187.9306) -> (-14.8723, 187.9448)
  line L1558 (-14.8723, 187.9448) -> (-14.591, 187.9306)
  line L1559 (-14.591, 187.9306) -> (-14.318, 187.889)
  line L1560 (-14.318, 187.889) -> (-14.0544, 187.8213)
  line L1561 (-14.0544, 187.8213) -> (-13.8017, 187.7288)
  line L1562 (-13.8017, 187.7288) -> (-13.5614, 187.613)
  line L1563 (-13.5614, 187.613) -> (-13.3346, 187.4752)
  line L1564 (-13.3346, 187.4752) -> (-13.1229, 187.3169)
  line L1565 (-13.1229, 187.3169) -> (-12.9277, 187.1393)
  line L1566 (-12.9277, 187.1393) -> (-12.7501, 186.9441)
  line L1567 (-12.7501, 186.9441) -> (-12.5918, 186.7324)
  line L1568 (-12.5918, 186.7324) -> (-12.4542, 186.5056)
  line L1569 (-12.4542, 186.5056) -> (-12.3383, 186.2653)
  line L1570 (-12.3383, 186.2653) -> (-12.2459, 186.0126)
  line L1571 (-12.2459, 186.0126) -> (-12.1781, 185.749)
  line L1572 (-12.1781, 185.749) -> (-12.1364, 185.476)
  line L1573 (-12.1364, 185.476) -> (-12.1223, 185.1949)
  line L1574 (-12.1223, 185.1949) -> (-12.1364, 184.9136)
  line L1575 (-12.1364, 184.9136) -> (-12.1781, 184.6406)
  line L1576 (-12.1781, 184.6406) -> (-12.2459, 184.377)
  line L1577 (-12.2459, 184.377) -> (-12.3383, 184.1243)
  line L1578 (-12.3383, 184.1243) -> (-12.4542, 183.884)
  line L1579 (-12.4542, 183.884) -> (-12.5918, 183.6574)
  line L1580 (-12.5918, 183.6574) -> (-12.7501, 183.4457)
  line L1581 (-12.7501, 183.4457) -> (-12.9277, 183.2503)
  line L1582 (-12.9277, 183.2503) -> (-13.1229, 183.0727)
  line L1583 (-13.1229, 183.0727) -> (-13.3346, 182.9144)
  line L1584 (-13.3346, 182.9144) -> (-13.5614, 182.7768)
  line L1585 (-13.5614, 182.7768) -> (-13.8017, 182.661)
  line L1586 (-13.8017, 182.661) -> (-14.0544, 182.5685)
  line L1587 (-14.0544, 182.5685) -> (-14.318, 182.5007)
  line L1588 (-14.318, 182.5007) -> (-14.591, 182.459)
  line L1589 (-14.591, 182.459) -> (-14.8723, 182.4448)
  line L1590 (-14.8723, 182.4448) -> (-15.1534, 182.459)
  line L1591 (-15.1534, 182.459) -> (-15.4264, 182.5007)
  line L1592 (-15.4264, 182.5007) -> (-15.69, 182.5685)
  line L1593 (-15.69, 182.5685) -> (-15.9427, 182.661)
  line L1594 (-15.9427, 182.661) -> (-16.183, 182.7768)
  line L1595 (-16.183, 182.7768) -> (-16.4099, 182.9144)
  line L1596 (-16.4099, 182.9144) -> (-16.6216, 183.0727)
  line L1597 (-16.6216, 183.0727) -> (-16.8167, 183.2503)
  line L1598 (-16.8167, 183.2503) -> (-16.9943, 183.4457)
  line L1599 (-16.9943, 183.4457) -> (-17.1526, 183.6574)
  line L1600 (-17.1526, 183.6574) -> (-17.2902, 183.884)
  line L1601 (-17.2902, 183.884) -> (-17.4062, 184.1243)
  line L1602 (-17.4062, 184.1243) -> (-17.4987, 184.377)
  line L1603 (-17.4987, 184.377) -> (-17.5664, 184.6406)
  line L1604 (-17.5664, 184.6406) -> (-17.6081, 184.9136)
  line L1605 (-17.6081, 184.9136) -> (-17.6222, 185.1949)
  line L1606 (-17.6222, 112.1968) -> (-17.6081, 112.4779)
  line L1607 (-17.6081, 112.4779) -> (-17.5664, 112.7511)
  line L1608 (-17.5664, 112.7511) -> (-17.4987, 113.0146)
  line L1609 (-17.4987, 113.0146) -> (-17.4062, 113.2672)
  line L1610 (-17.4062, 113.2672) -> (-17.2902, 113.5076)
  line L1611 (-17.2902, 113.5076) -> (-17.1526, 113.7343)
  line L1612 (-17.1526, 113.7343) -> (-16.9943, 113.9462)
  line L1613 (-16.9943, 113.9462) -> (-16.8167, 114.1415)
  line L1614 (-16.8167, 114.1415) -> (-16.6216, 114.3189)
  line L1615 (-16.6216, 114.3189) -> (-16.4099, 114.4771)
  line L1616 (-16.4099, 114.4771) -> (-16.183, 114.6149)
  line L1617 (-16.183, 114.6149) -> (-15.9427, 114.7306)
  line L1618 (-15.9427, 114.7306) -> (-15.69, 114.8233)
  line L1619 (-15.69, 114.8233) -> (-15.4264, 114.8908)
  line L1620 (-15.4264, 114.8908) -> (-15.1534, 114.9325)
  line L1621 (-15.1534, 114.9325) -> (-14.8723, 114.947)
  line L1622 (-14.8723, 114.947) -> (-14.591, 114.9325)
  line L1623 (-14.591, 114.9325) -> (-14.318, 114.8908)
  line L1624 (-14.318, 114.8908) -> (-14.0544, 114.8233)
  line L1625 (-14.0544, 114.8233) -> (-13.8017, 114.7306)
  line L1626 (-13.8017, 114.7306) -> (-13.5614, 114.6149)
  line L1627 (-13.5614, 114.6149) -> (-13.3346, 114.4771)
  line L1628 (-13.3346, 114.4771) -> (-13.1229, 114.3189)
  line L1629 (-13.1229, 114.3189) -> (-12.9277, 114.1415)
  line L1630 (-12.9277, 114.1415) -> (-12.7501, 113.9462)
  line L1631 (-12.7501, 113.9462) -> (-12.5918, 113.7343)
  line L1632 (-12.5918, 113.7343) -> (-12.4542, 113.5076)
  line L1633 (-12.4542, 113.5076) -> (-12.3383, 113.2672)
  line L1634 (-12.3383, 113.2672) -> (-12.2459, 113.0146)
  line L1635 (-12.2459, 113.0146) -> (-12.1781, 112.7511)
  line L1636 (-12.1781, 112.7511) -> (-12.1364, 112.4779)
  line L1637 (-12.1364, 112.4779) -> (-12.1223, 112.1968)
  line L1638 (-12.1223, 112.1968) -> (-12.1364, 111.9156)
  line L1639 (-12.1364, 111.9156) -> (-12.1781, 111.6425)
  line L1640 (-12.1781, 111.6425) -> (-12.2459, 111.3789)
  line L1641 (-12.2459, 111.3789) -> (-12.3383, 111.1264)
  line L1642 (-12.3383, 111.1264) -> (-12.4542, 110.8859)
  line L1643 (-12.4542, 110.8859) -> (-12.5918, 110.6592)
  line L1644 (-12.5918, 110.6592) -> (-12.7501, 110.4477)
  line L1645 (-12.7501, 110.4477) -> (-12.9277, 110.2524)
  line L1646 (-12.9277, 110.2524) -> (-13.1229, 110.0749)
  line L1647 (-13.1229, 110.0749) -> (-13.3346, 109.9165)
  line L1648 (-13.3346, 109.9165) -> (-13.5614, 109.7787)
  line L1649 (-13.5614, 109.7787) -> (-13.8017, 109.6629)
  line L1650 (-13.8017, 109.6629) -> (-14.0544, 109.5706)
  line L1651 (-14.0544, 109.5706) -> (-14.318, 109.5027)
  line L1652 (-14.318, 109.5027) -> (-14.591, 109.461)
  line L1653 (-14.591, 109.461) -> (-14.8723, 109.4469)
  line L1654 (-14.8723, 109.4469) -> (-15.1534, 109.461)
  line L1655 (-15.1534, 109.461) -> (-15.4264, 109.5027)
  line L1656 (-15.4264, 109.5027) -> (-15.69, 109.5706)
  line L1657 (-15.69, 109.5706) -> (-15.9427, 109.6629)
  line L1658 (-15.9427, 109.6629) -> (-16.183, 109.7787)
  line L1659 (-16.183, 109.7787) -> (-16.4099, 109.9165)
  line L1660 (-16.4099, 109.9165) -> (-16.6216, 110.0749)
  line L1661 (-16.6216, 110.0749) -> (-16.8167, 110.2524)
  line L1662 (-16.8167, 110.2524) -> (-16.9943, 110.4477)
  line L1663 (-16.9943, 110.4477) -> (-17.1526, 110.6592)
  line L1664 (-17.1526, 110.6592) -> (-17.2902, 110.8859)
  line L1665 (-17.2902, 110.8859) -> (-17.4062, 111.1264)
  line L1666 (-17.4062, 111.1264) -> (-17.4987, 111.3789)
  line L1667 (-17.4987, 111.3789) -> (-17.5664, 111.6425)
  line L1668 (-17.5664, 111.6425) -> (-17.6081, 111.9156)
  line L1669 (-17.6081, 111.9156) -> (-17.6222, 112.1968)
  line L1670 (68.0346, 112.1957) -> (68.0455, 112.4104)
  line L1671 (68.0455, 112.4104) -> (68.0772, 112.6191)
  line L1672 (68.0772, 112.6191) -> (68.129, 112.8203)
  line L1673 (68.129, 112.8203) -> (68.1996, 113.0133)
  line L1674 (68.1996, 113.0133) -> (68.288, 113.1969)
  line L1675 (68.288, 113.1969) -> (68.3932, 113.3698)
  line L1676 (68.3932, 113.3698) -> (68.5142, 113.5317)
  line L1677 (68.5142, 113.5317) -> (68.6496, 113.6806)
  line L1678 (68.6496, 113.6806) -> (68.7987, 113.8163)
  line L1679 (68.7987, 113.8163) -> (68.9605, 113.9372)
  line L1680 (68.9605, 113.9372) -> (69.1336, 114.0423)
  line L1681 (69.1336, 114.0423) -> (69.317, 114.1308)
  line L1682 (69.317, 114.1308) -> (69.5101, 114.2015)
  line L1683 (69.5101, 114.2015) -> (69.7113, 114.2531)
  line L1684 (69.7113, 114.2531) -> (69.9198, 114.2848)
  line L1685 (69.9198, 114.2848) -> (70.1346, 114.2959)
  line L1686 (70.1346, 114.2959) -> (70.3492, 114.2848)
  line L1687 (70.3492, 114.2848) -> (70.5578, 114.2531)
  line L1688 (70.5578, 114.2531) -> (70.759, 114.2015)
  line L1689 (70.759, 114.2015) -> (70.9519, 114.1308)
  line L1690 (70.9519, 114.1308) -> (71.1355, 114.0423)
  line L1691 (71.1355, 114.0423) -> (71.3087, 113.9372)
  line L1692 (71.3087, 113.9372) -> (71.4704, 113.8163)
  line L1693 (71.4704, 113.8163) -> (71.6194, 113.6806)
  line L1694 (71.6194, 113.6806) -> (71.755, 113.5317)
  line L1695 (71.755, 113.5317) -> (71.8759, 113.3698)
  line L1696 (71.8759, 113.3698) -> (71.9811, 113.1969)
  line L1697 (71.9811, 113.1969) -> (72.0695, 113.0133)
  line L1698 (72.0695, 113.0133) -> (72.1401, 112.8203)
  line L1699 (72.1401, 112.8203) -> (72.1918, 112.6191)
  line L1700 (72.1918, 112.6191) -> (72.2237, 112.4104)
  line L1701 (72.2237, 112.4104) -> (72.2345, 112.1957)
  line L1702 (72.2345, 112.1957) -> (72.2237, 111.9811)
  line L1703 (72.2237, 111.9811) -> (72.1918, 111.7727)
  line L1704 (72.1918, 111.7727) -> (72.1401, 111.5711)
  line L1705 (72.1401, 111.5711) -> (72.0695, 111.3782)
  line L1706 (72.0695, 111.3782) -> (71.9811, 111.1949)
  line L1707 (71.9811, 111.1949) -> (71.8759, 111.0216)
  line L1708 (71.8759, 111.0216) -> (71.755, 110.8601)
  line L1709 (71.755, 110.8601) -> (71.6194, 110.7109)
  line L1710 (71.6194, 110.7109) -> (71.4704, 110.5752)
  line L1711 (71.4704, 110.5752) -> (71.3087, 110.4546)
  line L1712 (71.3087, 110.4546) -> (71.1355, 110.3492)
  line L1713 (71.1355, 110.3492) -> (70.9519, 110.261)
  line L1714 (70.9519, 110.261) -> (70.759, 110.1903)
  line L1715 (70.759, 110.1903) -> (70.5578, 110.1383)
  line L1716 (70.5578, 110.1383) -> (70.3492, 110.1066)
  line L1717 (70.3492, 110.1066) -> (70.1346, 110.0956)
  line L1718 (70.1346, 110.0956) -> (69.9198, 110.1066)
  line L1719 (69.9198, 110.1066) -> (69.7113, 110.1383)
  line L1720 (69.7113, 110.1383) -> (69.5101, 110.1903)
  line L1721 (69.5101, 110.1903) -> (69.317, 110.261)
  line L1722 (69.317, 110.261) -> (69.1336, 110.3492)
  line L1723 (69.1336, 110.3492) -> (68.9605, 110.4546)
  line L1724 (68.9605, 110.4546) -> (68.7987, 110.5752)
  line L1725 (68.7987, 110.5752) -> (68.6496, 110.7109)
  line L1726 (68.6496, 110.7109) -> (68.5142, 110.8601)
  line L1727 (68.5142, 110.8601) -> (68.3932, 111.0216)
  line L1728 (68.3932, 111.0216) -> (68.288, 111.1949)
  line L1729 (68.288, 111.1949) -> (68.1996, 111.3782)
  line L1730 (68.1996, 111.3782) -> (68.129, 111.5711)
  line L1731 (68.129, 111.5711) -> (68.0772, 111.7727)
  line L1732 (68.0772, 111.7727) -> (68.0455, 111.9811)
  line L1733 (68.0455, 111.9811) -> (68.0346, 112.1957)
  line L1734 (82.035, 112.1957) -> (82.0458, 112.4104)
  line L1735 (82.0458, 112.4104) -> (82.0775, 112.6191)
  line L1736 (82.0775, 112.6191) -> (82.1294, 112.8203)
  line L1737 (82.1294, 112.8203) -> (82.2, 113.0133)
  line L1738 (82.2, 113.0133) -> (82.2883, 113.1969)